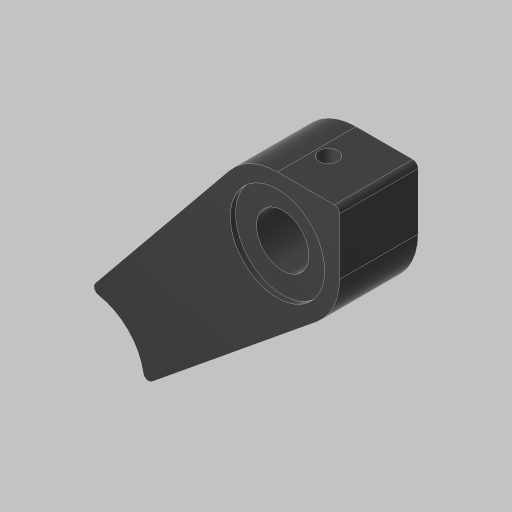
# Autodesk Inventor part: CL7-004
Saved by Autodesk Inventor 2023.5 (Build 275446000, 446)
## iProperties
Created: 2025-03-17
Part Number: CL7-004
Material: ABS Plastic
Document SubType Name: Modeling
Designer: dlangdon
Density: 1.06 g/cm^3
Appearance: Smooth - Black
Author: dlangdon
Autodesk Inventor part; units mm, degrees
ref_plane "YZ Plane" through (0, 0, 0) normal (1, 0, 0) x (0, 1, 0)
ref_plane "XZ Plane" through (0, 0, 0) normal (0, 1, 0) x (-1, 0, 0)
ref_plane "XY Plane" through (0, 0, 0) normal (0, 0, 1) x (1, 0, 0)
sketch "Sketch1" plane through (0, 0, 0) normal (0, 0, 1) x (1, 0, 0)
  line L0 (-76.2, 76.2) -> (76.2, 76.2) construction
  line L1 (76.2, 76.2) -> (76.2, -76.2) construction
  line L2 (76.2, -76.2) -> (-76.2, -76.2) construction
  line L3 (-76.2, -76.2) -> (-76.2, 76.2) construction
  line L4 (-76.2, 76.2) -> (76.2, -76.2) construction
  line L5 (76.2, 76.2) -> (-76.2, -76.2) construction
  circle A0 centre (-76.2, -76.2) radius 16.764 construction
  circle A1 centre (76.2, -76.2) radius 16.764 construction
  circle A2 centre (-19.05, -19.05) radius 7.9375
  circle A3 centre (19.05, -19.05) radius 7.9375 construction
  line L6 (-19.05, -19.05) -> (19.05, -19.05) construction
  circle A4 centre (-19.05, -19.05) radius 19.05 construction
  circle A5 centre (19.05, -19.05) radius 19.05 construction
  circle A6 centre (-19.05, -19.05) radius 18.796 construction
  circle A7 centre (19.05, -19.05) radius 18.796 construction
  arc A8 (-59.436, -76.2) -> (-76.2, -59.436) centre (-76.2, -76.2) ccw
  line L7 (-19.05, 0) -> (-3.4943, 0)
  line L8 (-33.6217, -7.1775) -> (-76.2, -59.436)
  line L9 (-7.1775, -33.6217) -> (-59.436, -76.2)
  line L10 (-19.05, -0.254) -> (-0.254, -0.254)
  line L11 (-0.254, -0.254) -> (-0.254, -19.05)
  arc A9 (-19.05, -0.254) -> (-33.6217, -7.1775) centre (-19.05, -19.05) ccw
  arc A10 (-7.1775, -33.6217) -> (-0.254, -19.05) centre (-19.05, -19.05) ccw
  point P0 (0, 0)
  point P1 (-33.1106, -7.4056)
  dimension "d0" = 152.4
  dimension "d1" = 152.4
  dimension "d2" = 33.528
  dimension "d3" = 15.875
  dimension "d4" = 38.1
  dimension "d7" = 0.254
  dimension "d8" = 0.254
  constraints: 24 end point, 12 point on circle, 10 centre point, 5 coincident, 5 horizontal, 4 point on line, 4 tangent, 2 equal radius, 2 midpoint, 2 parallel, 2 perpendicular, 1 vertical alignment, 4 other
  measures "d0" distance of L1.end L2.end
  measures "d1" distance of L0.end L1.end
  measures "d2" diameter of A0
  measures "d3" diameter of A2
  measures "d4" distance of L6.start L6.end
  measures "d8" radial gap between concentric circles of A5 A7
extrude "Extrusion1" add sketch "Sketch1" along normal mid plane 23.8125
fillet "Fillet1" radius 1.5875 3 edges at (-0.254, -0.254, 0) (-76.2, -59.436, 0) (-59.436, -76.2, 0)
sketch "Sketch2" plane through (0, 0, 11.9062) normal (0, 0, 1) x (1, 0, 0)
  circle A0 centre (-19.05, -19.05) radius 7.9375 projected
  circle A1 centre (-19.05, -19.05) radius 14.2875
  point P0 (0, 0)
  dimension "d12" = 28.575
  constraints: 1 centre point, 1 coincident
  measures "d12" diameter of A1
extrude "Extrusion2" cut sketch "Sketch2" against normal blind 1.5875
mirror "Mirror1" about plane through (0, 0, 0) normal (0, 0, 1) of "Extrusion2"
sketch "Sketch3" plane through (0, 0, 11.9062) normal (0, 0, 1) x (1, 0, 0)
  circle A0 centre (-19.05, -19.05) radius 14.2875 construction
  arc A1 (-59.6805, -73.3471) -> (-57.1134, -74.3077) centre (-58.1162, -73.077) ccw construction
  line L0 (-57.1134, -74.3077) -> (-7.1775, -33.6217) construction
  arc A2 (-7.1775, -33.6217) -> (-0.254, -19.05) centre (-19.05, -19.05) ccw construction
  line L1 (-0.254, -19.05) -> (-0.254, -1.8415) construction
  arc A3 (-0.254, -1.8415) -> (-1.8415, -0.254) centre (-1.8415, -1.8415) ccw construction
  line L2 (-1.8415, -0.254) -> (-19.05, -0.254) construction
  arc A4 (-19.05, -0.254) -> (-33.6217, -7.1775) centre (-19.05, -19.05) ccw construction
  line L3 (-33.6217, -7.1775) -> (-74.3077, -57.1134) construction
  arc A5 (-74.3077, -57.1134) -> (-73.3471, -59.6805) centre (-73.077, -58.1162) ccw construction
  arc A6 (-59.6805, -73.3471) -> (-73.3471, -59.6805) centre (-76.2, -76.2) ccw construction
  line L4 (19.05, 0) -> (-21.3612, -40.4112) construction
  line L5 (19.05, 0) -> (-21.3612, 40.4112) construction
  line L6 (19.05, 0) -> (0, 0) construction
  point P0 (-6.35, 0)
  dimension "d15" = 6.096
  dimension "d16" = 19.05
  dimension "d17" = 25.4
  dimension "d18" = 57.15
  dimension "d19" = 57.15
  dimension "d20" = 45
  constraints: 6 end point, 1 horizontal alignment, 1 perpendicular
  measures "d15" distance from line of L1 point (-6.35, 0)
  measures "d16" vertical distance of A0.centre point (-6.35, 0)
  measures "d17" distance of point (-6.35, 0) L4.start
  measures "d18" distance of L4.start L5.end
  measures "d19" distance of L4.start L4.end
  measures "d20" angle of L4 L6
ref_plane "Work Plane1" through (-0.719, -0.719, -11.9062) normal (-0.7071068, -0.7071068, 0) x (0.7071068, -0.7071068, 0)
sketch "Sketch5" plane through (-19.05, -0.254, 11.9062) normal (0, 1, 0) x (1, 0, 0)
  line L0 (18.796, 0) -> (18.796, 23.8125) construction
  line L1 (-14.5717, 0) -> (-14.5717, 23.8125) construction
  circle A0 centre (3.556, 11.9062) radius 2.875
  point P0 (19.05, 11.9062)
  point P1 (-14.5717, 11.9062)
  dimension "d28" = 15.24
  dimension "d29" = 5.75
  constraints: 1 centre point, 1 coincident, 1 horizontal alignment, 1 midpoint
  measures "d28" distance from line of L0 point (3.556, 11.906)
  measures "d29" diameter of A0
extrude "Extrusion3" cut sketch "Sketch5" against normal blind 7.62
equation "\"d7\" = d8"
equation "\"d19\" = d18"
body "Solid1"
